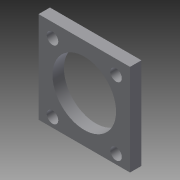
# Autodesk Inventor part: Ball grabber bearing mount
Saved by Autodesk Inventor 2013 (Build 170138000, 138)
## iProperties
Created: 2014-02-15
Part Number: Ball grabber bearing mount
Material: Generic
Document SubType Name: Modeling
Designer: robotics
Density: 1 g/cm^3
Author: robotics
Autodesk Inventor part; units mm, degrees
ref_plane "YZ Plane" through (0, 0, 0) normal (1, 0, 0) x (0, 1, 0)
ref_plane "XZ Plane" through (0, 0, 0) normal (0, 1, 0) x (-1, 0, 0)
ref_plane "XY Plane" through (0, 0, 0) normal (0, 0, 1) x (1, 0, 0)
sketch "Sketch1" plane through (0, 0, 0) normal (0, 0, 1) x (1, 0, 0)
  line L0 (0, 0) -> (50.8, 0)
  line L1 (50.8, 0) -> (50.8, 50.8)
  line L2 (50.8, 50.8) -> (0, 50.8)
  line L3 (0, 50.8) -> (0, 0)
  circle A0 centre (25.4, 25.4) radius 17.653
  line L4 (7.747, 7.747) -> (7.747, 43.053) construction
  line L5 (7.747, 43.053) -> (43.053, 43.053) construction
  line L6 (43.053, 43.053) -> (43.053, 5.1448) construction
  line L7 (43.053, 5.1448) -> (7.747, 5.1448) construction
  circle A1 centre (7.747, 43.053) radius 3.2004
  circle A2 centre (43.053, 43.053) radius 3.2004
  circle A3 centre (43.053, 5.1448) radius 3.2004
  circle A4 centre (7.747, 5.1448) radius 3.2004
  dimension "d0" = 50.8
  dimension "d1" = 50.8
  dimension "d2" = 35.306
  dimension "d3" = 6.4008
  dimension "d4" = 6.4008
  dimension "d5" = 6.4008
  dimension "d6" = 6.4008
  constraints: 16 end point, 5 centre point, 4 coincident, 4 parallel, 3 perpendicular, 1 horizontal
  measures "d0" distance of L2.end L1.end
  measures "d1" distance of L1.end L0.end
  measures "d2" diameter of A0
  measures "d3" diameter of A1
  measures "d4" diameter of A2
  measures "d5" diameter of A3
  measures "d6" diameter of A4
extrude "Extrusion1" add sketch "Sketch1" along normal blind 6.35
body "Solid1"
